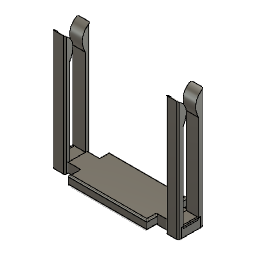
iphone tripod mount v1 (Autodesk Fusion 360 design; units mm, degrees)
Autodesk Fusion 360 part; units mm, degrees
sketch "Sketch1" plane through (0, 0, 0) normal (0, 1, 0) x (1, 0, 0) in component "Component"
  line L0 (25, -13) -> (-25, -13)
  line L1 (-25, -13) -> (-25, 13)
  line L2 (-25, 13) -> (25, 13)
  line L3 (25, 13) -> (25, -13)
  line L4 (25, -13) -> (-25, 13) construction
  line L5 (-25, -13) -> (25, 13) construction
  circle A0 centre (0, 0) radius 3.175
  line L6 (0, 6) -> (40, 6)
  line L7 (40, 6) -> (40, -6)
  line L8 (40, -6) -> (0, -6)
  line L9 (0, -6) -> (0, 6)
  line L10 (0, -20) -> (0, -2.5)
  line L11 (0, 6) -> (-40, 6)
  line L12 (-40, -6) -> (0, -6)
  line L13 (-40, 6) -> (-40, -6)
  line L14 (0, -6) -> (0, 6)
  dimension "d1" = 50
  dimension "d2" = 26
  dimension "d3" = 6.35
  dimension "d4" = 12
  dimension "d5" = 40
  constraint horizontal L0
  constraint perpendicular L0 L1
  constraint parallel L0 L2
  constraint parallel L1 L3
  constraint coincident L4 A0.centre
  constraint coincident L5 A0.centre
  constraint coincident A0.centre origin
  constraint horizontal L6
  constraint vertical L7
  constraint horizontal L8
  constraint vertical L9
  constraint coincident A0.centre L9
  constraint midpoint L9 A0.centre
  constraint symmetric L6.start L10 L9.end
  constraint symmetric L6.end L10 L11.end
  constraint symmetric L7.end L10 L12.start
  constraint symmetric L8.end L10 L9.start
  measures "d1" distance of L1.end L2.end
  measures "d2" distance of L0.end L1.end
  measures "d3" diameter of A0
  measures "d4" distance of L6.start L8.end
  measures "d5" distance of L6.start L6.end
extrude "Extrude1" add sketch "Sketch1" along normal blind 6 makes body 1 in component "Component"
extrude "Extrude2" cut sketch "Sketch1" along normal blind 4 contours A0 L9 L10 L14 | A0 L9 L10 L14 bodies 1 in component "Component"
thread "Thread1" "ANSI Unified Screw Threads 0.25 1/4-20 UNC 3B" major diameter 6.35 minor diameter 5.1156 pitch 1.27 angle 60 modelled right hand crest width 0.3725 on face at (3.1592, 1.3333, 0.3161) crest through (2.5578, 0.3175, 0) on bodies 1 in component "Component"
fillet "Fillet1" radius 1 11 edges at (0, 6, 13) (0, 6, -13) (-25, 6, -9.5) (-25, 6, 9.5) (25, 6, 9.5) (25, 6, -9.5) (0, 0, 13) (25, 0, 9.5) (25, 0, -9.5) (0, 0, -13) (-25, 0, -9.5) on bodies 1 in component "Component"
sketch "Sketch2" plane through (-40, 0, 0) normal (-1, 0, 0) x (0, 0, 1) in component "Component"
  line L0 (-6, 0) -> (6, 0)
  line L1 (6, 0) -> (6, 6)
  line L2 (-6, 6) -> (-6, 0)
  line L3 (0, 0) -> (8, 0)
  line L4 (8, 0) -> (8, 76)
  line L5 (0, 0) -> (0, 6)
  line L6 (8, 68.5) -> (3, 68.5)
  line L7 (5, 6) -> (5, 61)
  spline S0 degree 5 poles (5, 61) (4.8373, 61.2986) (4.5267, 61.8984) (4.105, 62.8057) (3.6325, 64.031) (3.2052, 65.5886) (2.9658, 67.169) (2.9496, 68.7637) (3.2004, 70.3547) (3.7663, 71.9121) (4.7004, 73.4004) (5.7849, 74.5077) (6.8082, 75.2785) (7.5867, 75.7642) (8, 76) knots 0 0 0 0 0 0 0.1 0.2 0.3 0.4 0.5 0.6 0.7 0.8 0.9 1 1 1 1 1 1
  line L8 (6.14, 74.9389) -> (9.86, 77.0611)
  line L9 (5, 6) -> (0, 6)
  line L10 (0, 1.75) -> (0, 22.5)
  line L11 (-5, 6) -> (-5, 61)
  line L12 (-8, 0) -> (-8, 76)
  spline S1 degree 5 poles (-5, 61) (-4.8373, 61.2986) (-4.5267, 61.8984) (-4.105, 62.8057) (-3.6325, 64.031) (-3.2052, 65.5886) (-2.9658, 67.169) (-2.9496, 68.7637) (-3.2004, 70.3547) (-3.7663, 71.9121) (-4.7004, 73.4004) (-5.7849, 74.5077) (-6.8082, 75.2785) (-7.5867, 75.7642) (-8, 76) knots 0 0 0 0 0 0 0.1 0.2 0.3 0.4 0.5 0.6 0.7 0.8 0.9 1 1 1 1 1 1
  line L13 (5.8267, 59.4834) -> (4.1733, 62.5166)
  line L14 (-5.8267, 59.4834) -> (-4.1733, 62.5166)
  line L15 (-6.14, 74.9389) -> (-9.86, 77.0611)
  line L16 (-5, 6) -> (0, 6)
  line L17 (0, 0) -> (0, 6)
  line L18 (0, 0) -> (-8, 0)
  point P0 (-3, 68.5)
  dimension "d10" = 8
  dimension "d11" = 76
  dimension "d12" = 5
  dimension "d13" = 7.5
  dimension "d14" = 15
  dimension "d15" = 5
  dimension "d16" = 55
  constraint coincident L3.start L5.start
  constraint perpendicular L1 L3
  constraint coincident L4 L6.start
  constraint perpendicular L4 L6
  constraint midpoint L4.end L8
  constraint perpendicular L5 L9
  constraint vertical L7
  constraint vertical L4
  constraint vertical L5
  constraint midpoint L7.end L13
  constraint symmetric L3.start L10 L5.start
  constraint symmetric L3.end L10 L12.start
  constraint symmetric L4.end L10 L12.end
  constraint symmetric L5.end L10 L9.end
  constraint symmetric L6.end L10 P0
  constraint symmetric L7.start L10 L11.start
  constraint symmetric L8.start L10 L15.start
  constraint symmetric L8.end L10 L15.end
  constraint symmetric L7.end L10 L11.end
  constraint symmetric L10 L13.start L14.start
  constraint symmetric L10 L13.end L14.end
  measures "d10" distance of L3.start L3.end
  measures "d11" distance of L3.end L4.end
  measures "d12" distance of L6.start L6.end
  measures "d13" distance of L4.end L6
  measures "d14" vertical distance of L4.end L7.end
  measures "d15" distance of L5.end L7.start
  measures "d16" distance of L7.start L7.end
extrude "Extrude3" add sketch "Sketch2" against normal blind 8 separate body makes body 2 in component "Component"
mirror "Mirror1" about plane through (0, 0, 0) normal (1, 0, 0) of bodies 2 makes body 3 in component "Component"
fillet "Fillet2" radius 1 10 edges at (-32, 38, -8) (-40, 38, -8) (-40, 6, 0) (-40, 38, 8) (-32, 38, 8) (32, 38, -8) (40, 38, -8) (32, 38, 8) (40, 38, 8) (40, 6, 0) on bodies 2 3 in component "Component"
component "Component" placed x (1, 0, 0) y (0, 1, 0) z (0, 0, 1) at (0, 0, 0)
equation "d14 = d13 * 2"
